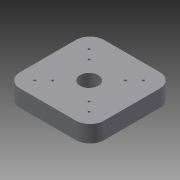
# Autodesk Inventor part: Part3
Saved by Autodesk Inventor 2015 (Build 190159000, 159)
## iProperties
Created: 2015-03-24
Part Number: Part3
Material: Generic
Document SubType Name: Modeling
Designer: nelsona
Density: 1 g/cm^3
Appearance: Default
Author: nelsona
Autodesk Inventor part; units mm, degrees
ref_plane "YZ Plane" through (0, 0, 0) normal (1, 0, 0) x (0, 1, 0)
ref_plane "XZ Plane" through (0, 0, 0) normal (0, 1, 0) x (-1, 0, 0)
ref_plane "XY Plane" through (0, 0, 0) normal (0, 0, 1) x (1, 0, 0)
sketch "Sketch1" plane through (0, 0, 0) normal (0, 1, 0) x (-1, 0, 0)
  line L0 (0, 0) -> (-38.1, 0)
  line L1 (-38.1, 0) -> (-38.1, -38.1)
  line L2 (-38.1, -38.1) -> (0, -38.1)
  line L3 (0, -38.1) -> (0, 0)
  dimension "d0" = 38.1
  dimension "d1" = 38.1
  constraints: 8 end point, 2 parallel, 1 horizontal, 1 perpendicular
  measures "d0" distance of L2.end L1.end
  measures "d1" distance of L1.end L0.end
extrude "Extrusion1" add sketch "Sketch1" along normal blind 7.62
sketch "Sketch2" plane through (0, 7.62, 0) normal (0, 1, 0) x (1, 0, 0)
  line L0 (4.5036, 33.196) -> (33.3072, 33.196)
  line L1 (33.3072, 33.196) -> (33.3072, 4.3924)
  line L2 (33.3072, 4.3924) -> (4.5036, 4.3924)
  line L3 (4.5036, 4.3924) -> (4.5036, 33.196)
  line L4 (33.3072, 33.196) -> (4.5036, 4.3924)
  line L5 (4.5036, 33.196) -> (33.3072, 4.3924)
  line L6 (18.9054, 18.7942) -> (27.1672, 27.056)
  line L7 (18.9054, 18.7942) -> (10.6436, 27.056)
  line L8 (18.9054, 18.7942) -> (10.6436, 10.5324)
  line L9 (18.9054, 18.7942) -> (27.1672, 10.5324)
  line L10 (18.9054, 18.7942) -> (31.2263, 31.1151)
  line L11 (18.9054, 18.7942) -> (6.5845, 31.1151)
  line L12 (18.9054, 18.7942) -> (6.5845, 6.4733)
  line L13 (18.9054, 18.7942) -> (31.2263, 6.4733)
  circle A0 centre (27.1672, 27.056) radius 0.508
  circle A1 centre (31.2263, 31.1151) radius 0.508
  circle A2 centre (6.5845, 31.1151) radius 0.508
  circle A3 centre (10.6436, 27.056) radius 0.508
  circle A4 centre (10.6436, 10.5324) radius 0.508
  circle A5 centre (6.5845, 6.4733) radius 0.508
  line L14 (18.9054, 18.7942) -> (27.1672, 10.5324)
  circle A6 centre (27.1672, 10.5324) radius 0.508
  circle A7 centre (31.2263, 6.4733) radius 0.508
  circle A8 centre (18.9054, 18.7942) radius 4.1783
  point P0 (0, 0)
  point P1 (27.2554, -7.62)
  dimension "d4" = 28.8036
  dimension "d5" = 28.8036
  dimension "d6" = 11.684
  dimension "d7" = 11.684
  dimension "d8" = 11.684
  dimension "d9" = 17.4244
  dimension "d10" = 17.4244
  dimension "d11" = 17.4244
  dimension "d12" = 17.4244
  dimension "d13" = 1.016
  dimension "d14" = 1.016
  dimension "d15" = 1.016
  dimension "d16" = 1.016
  dimension "d17" = 1.016
  dimension "d18" = 1.016
  dimension "d19" = 11.684
  dimension "d20" = 1.016
  dimension "d21" = 1.016
  dimension "d22" = 8.3566
  constraints: 30 end point, 9 centre point, 9 coincident, 8 point on line, 2 parallel, 1 collinear, 1 horizontal, 1 midpoint, 1 perpendicular
  measures "d4" distance of L1.end L2.end
  measures "d5" distance of L0.end L1.end
  measures "d6" distance of L6.start L6.end
  measures "d7" distance of L6.start L7.end
  measures "d8" distance of L6.start L8.end
  measures "d9" distance of L6.start L10.end
  measures "d10" distance of L6.start L11.end
  measures "d11" distance of L6.start L12.end
  measures "d12" distance of L6.start L13.end
  measures "d13" diameter of A0
  measures "d14" diameter of A1
  measures "d15" diameter of A2
  measures "d16" diameter of A3
  measures "d17" diameter of A4
  measures "d18" diameter of A5
  measures "d19" distance of L6.start L9.end
  measures "d20" diameter of A6
  measures "d21" diameter of A7
  measures "d22" diameter of A8
extrude "Extrusion2" cut sketch "Sketch2" against normal blind 25.4 contours A2 L5 | L5 A2 | A1 L4 | L4 A1 | A5 L4 | L4 A5 | A7 L5 | L5 A7 | A3 L5 | L5 A3 | A0 L4 | L4 A0 | A4 L4 | L4 A4 | A6 L5 | L5 A6 | A8 L4 L5 | L5 L4 A8 | A8 L5 L4 | L4 L5 A8
fillet "Fillet1" radius 6.35 4 edges at (38.1, 3.81, 0) (0, 3.81, 0) (0, 3.81, -38.1) (38.1, 3.81, -38.1)
body "Solid1"
